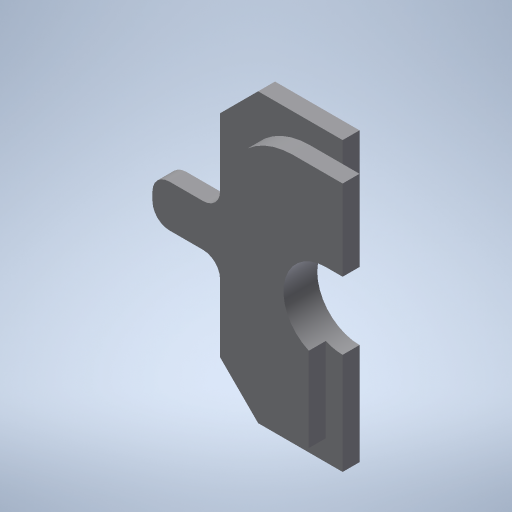
# Autodesk Inventor part: Chamber_lid
Saved by Autodesk Inventor 2023.3 (Build 273359000, 359)
## iProperties
Created: 2023-01-05
Part Number: Chamber_lid
Material: Generisch
Document SubType Name: Modeling
Designer: splath
Density: 1 g/cm^3
Appearance: Vorgabe
Author: splath
Autodesk Inventor part; units mm, degrees
ref_plane "YZ Plane" through (0, 0, 0) normal (1, 0, 0) x (0, 1, 0)
ref_plane "XZ Plane" through (0, 0, 0) normal (0, 1, 0) x (-1, 0, 0)
ref_plane "XY Plane" through (0, 0, 0) normal (0, 0, 1) x (1, 0, 0)
sketch "Sketch1" plane through (0, 0, 0) normal (0, 1, 0) x (-1, 0, 0)
  line L0 (-10, 17) -> (10, 17)
  line L1 (14.5, 12.5) -> (14.5, -12.5)
  line L2 (10, -17) -> (-10, -17)
  line L3 (-14.5, -12.5) -> (-14.5, 12.5)
  line L4 (-14.5, 17) -> (14.5, -17) construction
  line L5 (14.5, 17) -> (-14.5, -17) construction
  line L6 (10, 17) -> (14.5, 12.5)
  line L7 (14.5, -12.5) -> (10, -17)
  line L8 (-14.5, -12.5) -> (-10, -17)
  line L9 (-14.5, 12.5) -> (-10, 17)
  line L10 (14.5, 2.5) -> (22.5, 2.5)
  line L11 (22.5, 2.5) -> (22.5, -2.5)
  line L12 (22.5, -2.5) -> (14.5, -2.5)
  line L13 (14.5, -2.5) -> (14.5, 2.5)
  point P0 (0, 0)
  point P1 (14.5, 0)
  dimension "d0" = 29
  dimension "d1" = 34
  dimension "d2" = 4.5
  dimension "d3" = 4.5
  dimension "d4" = 4.5
  dimension "d5" = 4.5
  dimension "d6" = 4.5
  dimension "d7" = 4.5
  dimension "d8" = 4.5
  dimension "d9" = 4.5
  dimension "d32" = 8
  dimension "d33" = 5
  constraints: 28 end point, 9 point on line, 4 midpoint, 4 parallel, 2 horizontal, 2 perpendicular
  measures "d0" distance of L4.end L5.end
  measures "d1" distance of L5.start L4.end
  measures "d2" distance of L0.end L5.start
  measures "d3" distance of L1.start L5.start
  measures "d4" distance of L1.end L4.end
  measures "d5" distance of L2.start L4.end
  measures "d6" distance of L3.start L5.end
  measures "d7" distance of L2.end L5.end
  measures "d8" distance of L3.end L4.start
  measures "d9" distance of L0.start L4.start
  measures "d32" distance of L11.end L12.end
  measures "d33" distance of L10.end L11.end
extrude "Extrusion1" add sketch "Sketch1" along normal blind 2
sketch "Sketch2" plane through (0, 2, 0) normal (0, 1, 0) x (1, 0, 0)
  point P0 (0, 0)
  point P1 (0, 0)
  constraints: 1 coincident
hole "Hole1" at (0, 2, 0) direction (0, -1, 0) diameter 10 end through all
sketch "Sketch3" plane through (0, 0, 0) normal (0, -1, 0) x (1, 0, 0)
  line L0 (-3.85, -14.85) -> (3.85, -14.85)
  line L1 (12.35, -6.35) -> (12.35, 6.35)
  line L2 (3.85, 14.85) -> (-3.85, 14.85)
  line L3 (-12.35, 6.35) -> (-12.35, -6.35)
  line L4 (-12.35, -14.85) -> (12.35, 14.85) construction
  line L5 (12.35, -14.85) -> (-12.35, 14.85) construction
  arc A0 (12.35, 6.35) -> (3.85, 14.85) centre (3.85, 6.35) ccw
  arc A1 (-3.85, 14.85) -> (-12.35, 6.35) centre (-3.85, 6.35) ccw
  arc A2 (-12.35, -6.35) -> (-3.85, -14.85) centre (-3.85, -6.35) ccw
  arc A3 (3.85, -14.85) -> (12.35, -6.35) centre (3.85, -6.35) ccw
  circle A4 centre (0, 0) radius 5 projected
  dimension "d19" = 29.7
  dimension "d20" = 24.7
  dimension "d21" = 8.5
  constraints: 12 end point, 8 point on circle, 8 point on line, 8 tangent, 4 centre point, 3 equal radius, 2 midpoint, 2 parallel, 1 horizontal, 1 perpendicular
  measures "d19" distance between parallel lines of L0 L2
  measures "d20" distance between parallel lines of L3 L1
  measures "d21" radius of A0
extrude "Extrusion2" add sketch "Sketch3" along normal blind 2
sketch "Sketch4" plane through (0, 2, 0) normal (0, 1, 0) x (1, 0, 0)
  line L0 (0, 0) -> (18.9222, 0)
  line L1 (18.9222, 0) -> (18.9222, -20.1905)
  line L2 (18.9222, -20.1905) -> (0, -20.1905)
  line L3 (0, -20.1905) -> (0, 0)
  line L4 (18.9222, 0) -> (0, 0)
  line L5 (0, 0) -> (0, 23.1186)
  line L6 (0, 23.1186) -> (18.9222, 23.1186)
  line L7 (18.9222, 23.1186) -> (18.9222, 0)
  line L8 (0, 31.7804) -> (0, -28.8523) construction
  line L9 (-30.7844, 0) -> (27.2066, 0) construction
  line L10 (0, 0) -> (0, 0)
  line L11 (0, 0) -> (0, 5)
  line L12 (0, 5) -> (0, 5)
  line L13 (0, 5) -> (0, 0)
  circle A0 centre (0, 0) radius 5 construction
  dimension "d24" = 0
  dimension "d25" = 0
  constraints: 24 end point, 6 equal length, 3 horizontal, 3 perpendicular, 3 point on line, 1 collinear, 1 vertical alignment, 1 other
  measures "d24" distance between parallel lines of L8 L3
  measures "d25" distance between parallel lines of L8 L5
extrude "Extrusion3" cut sketch "Sketch4" against normal blind 2
sketch "Sketch5" plane through (0, 0, 0) normal (0, 1, 0) x (1, 0, 0)
  arc A0 (0, -5) -> (0, 5) centre (0, 0) ccw construction
  line L0 (0, -14.85) -> (0, -5) construction
  line L1 (0, -14.85) -> (3.85, -14.85) construction
  arc A1 (3.85, -14.85) -> (12.35, -6.35) centre (3.85, -6.35) ccw construction
  line L2 (12.35, -6.35) -> (12.35, 6.35) construction
  arc A2 (12.35, 6.35) -> (3.85, 14.85) centre (3.85, 6.35) ccw construction
  line L3 (3.85, 14.85) -> (0, 14.85) construction
  line L4 (2, 0) -> (15.8962, 0)
  line L5 (15.8962, 0) -> (15.8962, -16.8587)
  line L6 (15.8962, -16.8587) -> (2, -16.8587)
  line L7 (2, -16.8587) -> (2, 0)
  line L8 (16.9966, 0) -> (-2, 0)
  line L9 (-2, 0) -> (-2, 17.7139)
  line L10 (-2, 17.7139) -> (16.9966, 17.7139)
  line L11 (16.9966, 17.7139) -> (16.9966, 0)
  line L12 (0, 0) -> (2, 0)
  line L13 (2, 0) -> (2, -5)
  line L14 (2, -5) -> (0, -5)
  line L15 (0, -5) -> (0, 0)
  arc A3 (0, -5) -> (0, 5) centre (0, 0) ccw construction
  line L16 (0, 5) -> (0, 14.85) projected
  point P0 (2, 0)
  point P1 (15.8962, 0)
  point P2 (0, 0)
  dimension "d30" = 2
  dimension "d31" = 2
  constraints: 24 end point, 6 parallel, 3 horizontal, 3 perpendicular, 1 point on circle, 1 point on line
  measures "d30" distance between parallel lines of L15 L9
  measures "d31" distance between parallel lines of L13 L15
extrude "Extrusion4" cut sketch "Sketch5" against normal blind 2
fillet "Fillet1" radius 2 4 edges at (-14.5, 1, 2.5) (-14.5, 1, -2.5) (-22.5, 1, 2.5) (-22.5, 1, -2.5)
thicken "Thicken1" operation cut thickness 0.3 both sides no extend neighbours no toward (0, 0, -1) faces at (-0.6167, -1.3333, 14.85) (-10.0809, -1.3333, 12.1315) (-12.35, -0.6667, 2.1167) (-4.4852, -1.3333, -14.8262) (-3.2333, -0.6667, -14.85)
equation "\"d3\" = d2"
equation "\"d4\" = d2"
equation "\"d5\" = d4"
equation "\"d6\" = d2"
equation "\"d7\" = d6"
equation "\"d8\" = d2"
equation "\"d9\" = d8"
equation "\"d31\" = d30"
body "Solid1"
